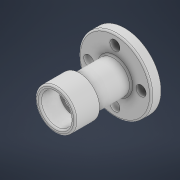
# Autodesk Inventor part: Pieza de practica 2
Saved by Autodesk Inventor 2022 (Build 260153000, 153)
## iProperties
Created: 2022-06-06
Part Number: Pieza de practica 2
Material: Genérico
Document SubType Name: Modeling
Designer: aleon
Density: 1 g/cm^3
Appearance: Valor por defecto
Author: aleon
Autodesk Inventor part; units mm, degrees
ref_plane "YZ Plane" through (0, 0, 0) normal (1, 0, 0) x (0, 1, 0)
ref_plane "XZ Plane" through (0, 0, 0) normal (0, 1, 0) x (-1, 0, 0)
ref_plane "XY Plane" through (0, 0, 0) normal (0, 0, 1) x (1, 0, 0)
sketch "Boceto1" plane through (0, 0, 0) normal (1, 0, 0) x (0, 1, 0)
  line L0 (25, 5.601225) -> (19, 5.601225)
  line L1 (19, 5.601225) -> (19, -18.398775)
  line L2 (19, -18.398775) -> (15, -18.398775)
  line L3 (15, -18.398775) -> (15, -80.798775)
  line L4 (15, -80.798775) -> (45, -80.798775)
  line L5 (45, -80.798775) -> (45, -68.598775)
  line L6 (45, -68.598775) -> (20, -68.598775)
  line L7 (20, -68.598775) -> (20, -24.398775)
  line L8 (20, -24.398775) -> (25, -24.398775)
  line L9 (25, -24.398775) -> (25, 5.601225)
  line L10 (0, 0) -> (0, 11.507163) construction
  line L11 (-25, 5.601225) -> (-19, 5.601225)
  line L12 (-19, 5.601225) -> (-19, -18.398775)
  line L13 (-19, -18.398775) -> (-15, -18.398775)
  line L14 (-15, -18.398775) -> (-15, -80.798775)
  line L15 (-15, -80.798775) -> (-45, -80.798775)
  line L16 (-45, -80.798775) -> (-45, -68.598775)
  line L17 (-45, -68.598775) -> (-20, -68.598775)
  line L18 (-20, -68.598775) -> (-20, -24.398775)
  line L19 (-20, -24.398775) -> (-25, -24.398775)
  line L20 (-25, -24.398775) -> (-25, 5.601225)
  dimension "d0" = 30
  dimension "d1" = 40
  dimension "d2" = 90
  dimension "d3" = 38
  dimension "d4" = 50
  dimension "d5" = 24
  dimension "d6" = 6
  dimension "d7" = 44.2
  dimension "d8" = 12.2
  constraints: 44 end point, 10 symmetric about line, 9 perpendicular, 1 horizontal, 1 vertical
  measures "d0" distance between parallel lines of L14 L3
  measures "d1" distance between parallel lines of L18 L7
  measures "d2" distance between parallel lines of L16 L5
  measures "d3" distance between parallel lines of L1 L12
  measures "d4" distance between parallel lines of L20 L9
  measures "d5" distance between parallel lines of L2 L11
  measures "d6" distance between parallel lines of L8 L13
  measures "d7" distance between parallel lines of L6 L8
  measures "d8" distance between parallel lines of L6 L15
sketch "Boceto1 outline for Revolución1" plane through (0, 0, 0) normal (1, 0, 0) x (0, 1, 0)
  line L0 (-25, 5.601225) -> (-25, -24.398775)
  line L1 (-19, 5.601225) -> (-25, 5.601225)
  line L2 (-19, -18.398775) -> (-19, 5.601225)
  line L3 (-15, -18.398775) -> (-19, -18.398775)
  line L4 (-15, -80.798775) -> (-15, -18.398775)
  line L5 (-45, -80.798775) -> (-15, -80.798775)
  line L6 (-45, -68.598775) -> (-45, -80.798775)
  line L7 (-20, -68.598775) -> (-45, -68.598775)
  line L8 (-20, -24.398775) -> (-20, -68.598775)
  line L9 (-25, -24.398775) -> (-20, -24.398775)
  line L10 (25, 5.601225) -> (19, 5.601225)
  line L11 (25, -24.398775) -> (25, 5.601225)
  line L12 (20, -24.398775) -> (25, -24.398775)
  line L13 (20, -68.598775) -> (20, -24.398775)
  line L14 (45, -68.598775) -> (20, -68.598775)
  line L15 (45, -80.798775) -> (45, -68.598775)
  line L16 (15, -80.798775) -> (45, -80.798775)
  line L17 (15, -18.398775) -> (15, -80.798775)
  line L18 (19, -18.398775) -> (15, -18.398775)
  line L19 (19, 5.601225) -> (19, -18.398775)
revolve "Revolución1" add sketch "Boceto1 outline for Revolución1" angle 360 about axis through (0, 0, 0) along (0, 0, 1)
sketch "Boceto4" plane through (0, 0, -68.598775) normal (0, 0, 1) x (1, 0, 0)
  circle A0 centre (0, -32.5) radius 6.25
  circle A1 centre (0, 32.5) radius 6.25
  circle A2 centre (-32.5, 0) radius 6.25
  circle A3 centre (32.5, 0) radius 6.25
  circle A4 centre (0, -32.5) radius 6.25
  circle A5 centre (0, 32.5) radius 6.25
  circle A6 centre (32.5, 0) radius 6.25
  circle A7 centre (-32.5, 0) radius 6.25
  point P0 (0, 0)
  dimension "d18" = 12.5
  dimension "d19" = 12.5
  dimension "d20" = 65
  dimension "d21" = 32.5
  dimension "d24" = 360
  constraints: 8 centre point, 17 other
  measures "d18" diameter of A0
  measures "d19" diameter of A1
  measures "d20" distance of A0.centre A1.centre
  measures "d21" distance of point (0, 0) A0.centre
sketch "Boceto4 outline for Extrusión1" plane through (0, 0, -68.598775) normal (0, 0, 1) x (1, 0, 0)
  circle A0 centre (-32.5, 0) radius 6.25
  circle A1 centre (0, -32.5) radius 6.25
  circle A2 centre (32.5, 0) radius 6.25
  circle A3 centre (0, 32.5) radius 6.25
extrude "Extrusión1" cut sketch "Boceto4 outline for Extrusión1" against normal through all
chamfer "Chaflán1" distance 3 distance2 3.5 1 edges at (0, 15, -80.7988) measured on face at (2.4062, -14.8058, -59.9988)
fillet "Empalme1" radius 2 4 edges at (0, 45, -68.5988) (0, 20, -68.5988) (0, 25, 5.6012) (0, 19, 5.6012)
